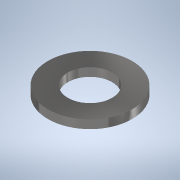
# Autodesk Inventor part: washer_m8
Saved by Autodesk Inventor 2020 (Build 240168000, 168)
## iProperties
Created: 2016-11-12
Part Number: washer_m8
Material: Generic
Document SubType Name: Modeling
Designer: jous
Density: 1 g/cm^3
Appearance: Default
Mass: 0.233031 g
Surface Area: 4.13936 cm^2
Volume: 0.233031 cm^3
Author: jous
Autodesk Inventor part; units mm, degrees
ref_plane "YZ Plane" through (0, 0, 0) normal (1, 0, 0) x (0, 1, 0)
ref_plane "XZ Plane" through (0, 0, 0) normal (0, 1, 0) x (-1, 0, 0)
ref_plane "XY Plane" through (0, 0, 0) normal (0, 0, 1) x (1, 0, 0)
sketch "Sketch1" plane through (0, 0, 0) normal (0, 0, 1) x (1, 0, 0)
  circle A0 centre (0, 0) radius 4.2
  circle A1 centre (0, 0) radius 8
  dimension "d0" = 8.4
  dimension "d1" = 16
  constraints: 2 centre point, 2 coincident
  measures "d0" diameter of A0
  measures "d1" diameter of A1
extrude "Extrusion1" add sketch "Sketch1" along normal blind 1.6
body "Solid1"
